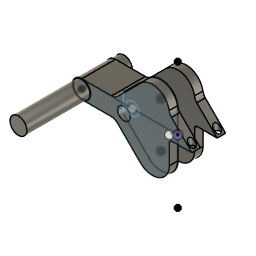
wrist-link (Autodesk Fusion 360 design; units mm, degrees)
Autodesk Fusion 360 part; units mm, degrees
sketch "Sketch2" plane through (0, 0, 0) normal (0, 1, 0) x (1, 0, 0)
  line L0 (0, 0) -> (0, -5.3431)
  line L1 (0, 0) -> (-15, 0)
  line L2 (0, 0) -> (0, 5.3431)
  line L3 (-6.8284, 8.1716) -> (-12.8787, 2.1213)
  line L4 (-12.8787, -2.1213) -> (-6.8284, -8.1716)
  arc A0 (-6.8284, -8.1716) -> (0, -5.3431) centre (-4, -5.3431) ccw
  arc A1 (0, 5.3431) -> (-6.8284, 8.1716) centre (-4, 5.3431) ccw
  circle A2 centre (-10.7574, 0) radius 1.5
  line L5 (-12.8787, -2.1213) -> (-12.8787, 2.1213)
  point P0 (0, -15)
  point P1 (0, 15)
  dimension "d2" = 15
  dimension "d3" = 15
  dimension "d4" = 15
  dimension "d5" = 4
  dimension "d6" = 4
  dimension "d23" = 3
  constraint vertical L0
  constraint coincident L0.start L1.start
  constraint perpendicular L0 L1
  constraint perpendicular L1 L2
  constraint coincident P0 L0
  constraint coincident P0 L4
  constraint tangent L0 A0
  constraint tangent L4 A0
  constraint coincident P1 L2
  constraint coincident P1 L3
  constraint tangent L2 A1
  constraint tangent L3 A1
  constraint coincident L1.end L4
  constraint coincident L1.end L3
  constraint perpendicular L1 L5
  measures "d2" distance of L0.start P0
  measures "d3" distance of L0.start L1.end
  measures "d4" distance of L0.start P1
  measures "d5" radius of A0
  measures "d6" radius of A1
  measures "d23" diameter of A2
ref_plane "WorkPlane1" through (0, 0, 0) normal (0, 1, 0) x (0, 0, 1)
ref_plane "WorkPlane2" through (0, 4, 0) normal (0, 1, 0) x (0, 0, 1)
sketch "Sketch4" plane through (0, 4, 0) normal (0, 1, 0) x (1, 0, 0)
  line L0 (0, 0) -> (0, -5.3431)
  line L1 (0, 0) -> (0, 5.3431)
  line L2 (0, 0) -> (-15, 0)
  line L3 (-6.8284, -8.1716) -> (-12.8787, -2.1213)
  line L4 (-6.8284, 8.1716) -> (-12.8787, 2.1213)
  arc A0 (-6.8284, -8.1716) -> (0, -5.3431) centre (-4, -5.3431) ccw
  arc A1 (0, 5.3431) -> (-6.8284, 8.1716) centre (-4, 5.3431) ccw
  circle A2 centre (-10.7574, 0) radius 1.5
  line L5 (-12.8787, -2.1213) -> (-12.8787, 2.1213)
  point P0 (0, -15)
  point P1 (0, 15)
  dimension "d12" = 15
  dimension "d13" = 15
  dimension "d14" = 15
  dimension "d15" = 4
  dimension "d16" = 4
  dimension "d20" = 3
  constraint coincident L0.start L1.start
  constraint vertical L0
  constraint parallel L0 L1
  constraint perpendicular L0 L2
  constraint coincident P0 L0
  constraint coincident P0 L3
  constraint tangent L0 A0
  constraint tangent L3 A0
  constraint coincident P1 L1
  constraint coincident P1 L4
  constraint tangent L1 A1
  constraint tangent L4 A1
  constraint coincident L2.end L3
  constraint coincident L2.end L4
  constraint vertical L5
  measures "d12" distance of L0.start P0
  measures "d13" distance of L0.start P1
  measures "d14" distance of L0.start L2.end
  measures "d15" radius of A0
  measures "d16" radius of A1
  measures "d20" diameter of A2
extrude "Extrude3" add sketch "Sketch4" along normal blind 2 contours L2 A2 | L2 A2 makes body 1
extrude "Extrude4" add sketch "Sketch2" against normal blind 2 separate body contours L0 L1 L4 A0 A2 L5 | L1 L2 L3 A1 A2 L5 makes body 2
sketch "Sketch7" plane through (0, 0, 0) normal (1, 0, 0) x (0, 1, 0)
  line L0 (0, 0) -> (0, 1)
  line L1 (0, 1) -> (-2, 1)
  dimension "d30" = 1
  constraint coincident L0.start origin
  constraint vertical L0
  constraint perpendicular L0 L1
  measures "d30" distance of L0.start L0.end
sketch "Sketch10" plane through (0, 0, 0) normal (0, 1, 0) x (1, 0, 0)
  line L0 (5.3431, 0) -> (0, -5.3431)
  line L1 (5.3431, 0) -> (11.5711, 0) construction
  line L2 (5.3431, 0) -> (0, 0)
  line L3 (0, 0) -> (0, -5.3431)
  point P0 (0, -5.3431)
  dimension "d34" = 135
  constraint horizontal L1
  constraint parallel L1 L2
  constraint perpendicular L2 L3
  constraint coincident L2.end L3.start
  constraint coincident P0 L0.end
  measures "d34" angle of L0 L1
extrude "Extrude6" add sketch "Sketch10" against normal blind 2 bodies 2
fillet "Fillet1" radius 2 1 edges at (0, -1, 5.3431) on bodies 2
sketch "Sketch11" plane through (0, 0, 0) normal (0, 0, -1) x (1, 0, 0)
  line L0 (0, 0) -> (5.3431, 0)
  line L1 (5.3431, 0) -> (5.3431, 2)
  line L2 (5.3431, 2) -> (0, 2)
  line L3 (0, 2) -> (0, 0)
  circle A0 centre (4.3431, 1) radius 0.75
  dimension "d41" = 1.5
  dimension "d42" = 1
  dimension "d43" = 1
  measures "d41" diameter of A0
  measures "d42" distance of L1 A0.centre
  measures "d43" distance of L2 A0.centre
extrude "Extrude7" cut sketch "Sketch11" against normal blind 2.5 contours A0 bodies 2
fillet "Fillet2" radius 0.5 1 edges at (0, -1, 0) on bodies 2
ref_plane "WorkPlane3" through (0, 2, 0) normal (0, 1, 0) x (0, 0, 1)
mirror "Mirror1" about plane through (0, 2, 0) normal (0, 1, 0) of bodies 2 makes body 3
extrude "Extrude9" cut sketch "Sketch4" along normal blind 2 contours L2 A2 | L2 A2 bodies 1
sketch "Sketch13" plane through (-12.8787, 0, 0) normal (-1, 0, 0) x (0, -1, 0)
  line L0 (-4, -2.1213) -> (-4, 2.1213)
  line L1 (-4, 2.1213) -> (-6, 2.1213)
  line L2 (-6, 2.1213) -> (-6, -2.1213)
  line L3 (-6, -2.1213) -> (-4, -2.1213)
  line L4 (-6, 2.1213) -> (2, 2.1213)
  line L5 (2, 2.1213) -> (2, -2.1213)
  line L6 (2, -2.1213) -> (-6, -2.1213)
  line L7 (-6, 2.1213) -> (-6, -2.1213)
  point P0 (2, 2.1213)
  constraint coincident L1.end L2.start
  constraint perpendicular L0 L4
  constraint perpendicular L4 L5
  constraint coincident L2.end L3.start
  constraint parallel L4 L6
  constraint coincident P0 L4.end
extrude "Extrude10" add sketch "Sketch13" along normal blind 10 bodies 1 2 3
fillet "Fillet3" radius 2 4 edges at (-12.8787, -1, -2.1213) (-12.8787, 5, -2.1213) (-12.8787, -1, 2.1213) (-12.8787, 5, 2.1213) on bodies 1
sketch "Sketch16" plane through (0, -2, 0) normal (0, -1, 0) x (1, 0, 0)
  circle A0 centre (-10.7574, 0) radius 1.5
  arc A1 (-0.0448, 5.9402) -> (-6.8284, 8.1716) centre (-4, 5.3431) ccw
  line L0 (-6.8284, 8.1716) -> (-12.2929, 2.7071)
  arc A2 (-13.7071, 2.1213) -> (-12.2929, 2.7071) centre (-13.7071, 4.1213) ccw
  line L1 (-13.7071, 2.1213) -> (-22.8787, 2.1213)
  line L2 (-22.8787, 2.1213) -> (-22.8787, -2.1213)
  line L3 (-22.8787, -2.1213) -> (-13.7071, -2.1213)
  arc A3 (-12.2929, -2.7071) -> (-13.7071, -2.1213) centre (-13.7071, -4.1213) ccw
  line L4 (-12.2929, -2.7071) -> (-6.8284, -8.1716)
  arc A4 (-6.8284, -8.1716) -> (0, -5.3431) centre (-4, -5.3431) ccw
  line L5 (0, -5.3431) -> (0, -0.5)
  arc A5 (0.5, 0) -> (0, -0.5) centre (0.5, -0.5) ccw
  line L6 (0.5, 0) -> (5.3431, 0)
  line L7 (5.3431, 0) -> (0.5186, 4.8246)
  arc A6 (-0.0448, 5.9402) -> (0.5186, 4.8246) centre (1.9328, 6.2388) ccw
  circle A7 centre (-20.7574, 0) radius 2.1213
  circle A8 centre (-20.7574, 0) radius 2
  dimension "d64" = 4
  constraint tangent L1 A7
  constraint tangent L2 A7
  constraint tangent L3 A7
  constraint concentric A7 A8
  measures "d64" diameter of A8
extrude "Extrude11" cut sketch "Sketch16" against normal blind 9 contours L1 L2 A7 | L2 L3 A7 bodies 1
extrude "Extrude12" cut sketch "Sketch16" against normal blind 9 contours A8 bodies 1
sketch "Sketch17" plane through (0, 0, 0) normal (0, 1, 0) x (1, 0, 0)
  circle A0 centre (15, 0) radius 2
  dimension "d67" = 4
  measures "d67" diameter of A0
extrude "Extrude13" add sketch "Sketch17" along normal blind 25 separate body makes body 4
copy_body "Body->Comp4" bodies 4 removing the originals makes body 5 in component "Component"
component "Component" placed x (1, 0, 0) y (0, 1, 0) z (0, 0, 1) at (-35.7574, -17, 0)
